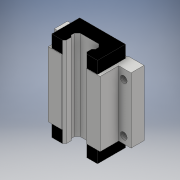
# Autodesk Inventor part: PATINS TRILHO LINEAR 15MM DFH-A_AL
Saved by Autodesk Inventor 2018 (Build 220112000, 112)
## iProperties
Created: 2018-09-22
Part Number: PATINS TRILHO LINEAR 15MM DFH-A_AL
Material: Genérico
Document SubType Name: Modeling
Designer: Usuario
Density: 1 g/cm^3
Appearance: Padrão
Author: Usuario
Autodesk Inventor part; units mm, degrees
ref_plane "YZ Plane" through (0, 0, 0) normal (1, 0, 0) x (0, 1, 0)
ref_plane "XZ Plane" through (0, 0, 0) normal (0, 1, 0) x (-1, 0, 0)
ref_plane "XY Plane" through (0, 0, 0) normal (0, 0, 1) x (1, 0, 0)
sketch "Esboço1" plane through (0, 0, 0) normal (0, 0, 1) x (1, 0, 0)
  line L0 (1.0341, 28.7122) -> (1.0341, -32.1101) construction
  line L1 (1.0341, 7.7011) -> (-4.7241, 7.7011)
  line L2 (-4.7241, 7.7011) -> (-6.4659, 5.9592)
  line L3 (-6.4659, 5.9592) -> (-6.4659, 3.9592)
  line L4 (-6.4659, 3.9592) -> (-5.2631, 2.7564)
  line L5 (-5.2631, 2.7564) -> (-5.2631, -0.2436)
  line L6 (-5.2631, -0.2436) -> (-6.4659, -1.4465)
  line L7 (-6.4659, -1.4465) -> (-6.4659, -1.6989)
  line L8 (-6.4659, -6.2989) -> (1.0341, -6.2989) construction
  line L9 (-22.4659, 9.7011) -> (-22.4659, 17.7011)
  line L10 (-17.9659, 24.9392) -> (-17.9659, -12.707) construction
  line L11 (-20.4659, 24.9392) -> (-20.4659, -12.707) construction
  line L12 (-15.4659, 24.9392) -> (-15.4659, -12.9196) construction
  line L13 (1.0341, 9.7011) -> (-29.6062, 9.7011) construction
  line L14 (-22.4659, 9.7011) -> (-14.8619, 9.7011)
  line L15 (-14.8619, 9.7011) -> (-14.8619, -1.6989)
  line L16 (1.0341, 16.4633) -> (-13.4863, 16.4633) construction
  line L17 (-13.4863, 16.4633) -> (-13.4863, -1.6989) construction
  arc A0 (-14.8619, -1.6989) -> (-22.4659, 9.7011) centre (-28.6186, -2.6389) ccw construction
  line L18 (-6.4659, -1.6989) -> (-6.4659, -6.2989) construction
  line L19 (-6.4659, -1.6989) -> (-14.8619, -1.6989)
  line L20 (-13.4863, 17.7011) -> (-12.9262, 17.1409)
  line L21 (-12.9262, 17.1409) -> (-5.8645, 17.1409)
  line L22 (-5.8645, 17.1409) -> (-5.3043, 17.7011)
  line L23 (-22.4659, 17.7011) -> (-13.4863, 17.7011)
  line L24 (-5.3043, 17.7011) -> (1.0341, 17.7011)
  line L25 (1.0341, 7.7011) -> (6.7923, 7.7011)
  line L26 (6.7923, 7.7011) -> (8.5341, 5.9592)
  line L27 (8.5341, 5.9592) -> (8.5341, 3.9592)
  line L28 (8.5341, 3.9592) -> (7.3313, 2.7564)
  line L29 (7.3313, 2.7564) -> (7.3313, -0.2436)
  line L30 (7.3313, -0.2436) -> (8.5341, -1.4465)
  line L31 (8.5341, -1.4465) -> (8.5341, -1.6989)
  line L32 (8.5341, -6.2989) -> (1.0341, -6.2989) construction
  line L33 (24.5341, 9.7011) -> (24.5341, 17.7011)
  line L34 (20.0341, 24.9392) -> (20.0341, -12.707) construction
  line L35 (22.5341, 24.9392) -> (22.5341, -12.707) construction
  line L36 (17.5341, 24.9392) -> (17.5341, -12.9196) construction
  line L37 (1.0341, 9.7011) -> (31.6744, 9.7011) construction
  line L38 (24.5341, 9.7011) -> (16.9301, 9.7011)
  line L39 (16.9301, 9.7011) -> (16.9301, -1.6989)
  line L40 (1.0341, 16.4633) -> (15.5546, 16.4633) construction
  line L41 (15.5546, 16.4633) -> (15.5546, -1.6989) construction
  arc A1 (24.5341, 9.7011) -> (16.9301, -1.6989) centre (30.6868, -2.6389) ccw construction
  line L42 (8.5341, -1.6989) -> (8.5341, -6.2989) construction
  line L43 (8.5341, -1.6989) -> (16.9301, -1.6989)
  line L44 (15.5546, 17.7011) -> (14.9944, 17.1409)
  line L45 (14.9944, 17.1409) -> (7.9327, 17.1409)
  line L46 (7.9327, 17.1409) -> (7.3725, 17.7011)
  line L47 (24.5341, 17.7011) -> (15.5546, 17.7011)
  line L48 (7.3725, 17.7011) -> (1.0341, 17.7011)
  dimension "d11" = 45
  dimension "d12" = 3
  dimension "d13" = 14
  dimension "d14" = 2
  dimension "d15" = 7.5
  dimension "d19" = 23.5
  dimension "d21" = 2.5
  dimension "d22" = 2.5
  dimension "d23" = 19
  constraints: 98 end point, 26 symmetric about line, 15 point on line, 9 perpendicular, 5 horizontal, 5 vertical, 4 point on circle, 2 centre point, 2 parallel, 1 other
  measures "d11" angle of L2 L1
  measures "d12" distance of L4.end L5.end
  measures "d13" distance between parallel lines of L8 L1
  measures "d14" distance of L2.end L3.end
  measures "d15" distance of L8.start L8.end
  measures "d19" distance of L9.end L24.end
  measures "d21" distance between parallel lines of L12 L10
  measures "d22" distance between parallel lines of L10 L11
  measures "d23" distance between parallel lines of L10 L0
extrude "Extrusão2" add sketch "Esboço1" along normal blind 40
sketch "Esboço2" plane through (0, 0, 40) normal (0, 0, 1) x (1, 0, 0)
  line L0 (-13.0314, -1.4465) -> (-13.0314, 15.7348)
  line L1 (-13.0314, 15.7348) -> (15.0996, 15.7348)
  line L2 (15.0996, 15.7348) -> (15.0996, -1.4465)
  line L3 (-6.4659, -1.4465) -> (-5.2631, -0.2436) projected
  line L4 (-6.4659, -1.4465) -> (-5.2631, -0.2436)
  line L5 (-5.2631, 2.7564) -> (-6.4659, 3.9592) projected
  line L6 (-5.2631, -0.2436) -> (-5.2631, 2.7564)
  line L7 (-5.2631, 2.7564) -> (-6.4659, 3.9592)
  line L8 (-6.4659, 3.9592) -> (-6.4659, 5.9592) projected
  line L9 (-6.4659, 3.9592) -> (-6.4659, 5.9592)
  line L10 (-6.4659, 5.9592) -> (-4.7241, 7.7011) projected
  line L11 (-6.4659, 5.9592) -> (-4.7241, 7.7011)
  line L12 (-4.7241, 7.7011) -> (6.7923, 7.7011) projected
  line L13 (-4.7241, 7.7011) -> (6.7923, 7.7011)
  line L14 (6.7923, 7.7011) -> (8.5341, 5.9592) projected
  line L15 (6.7923, 7.7011) -> (8.5341, 5.9592)
  line L16 (8.5341, 3.9592) -> (8.5341, 5.9592) projected
  line L17 (8.5341, 5.9592) -> (8.5341, 3.9592)
  line L18 (7.3313, -0.2436) -> (7.3313, 2.7564) projected
  line L19 (8.5341, 3.9592) -> (7.3313, 2.7564)
  line L20 (7.3313, 2.7564) -> (7.3313, -0.2436)
  line L21 (8.5341, -1.4465) -> (7.3313, -0.2436) projected
  line L22 (7.3313, -0.2436) -> (8.5341, -1.4465)
  line L23 (15.0996, -1.4465) -> (8.5341, -1.4465)
  line L24 (-6.4659, -1.4465) -> (-13.0314, -1.4465)
  constraints: 32 end point, 7 collinear, 4 parallel, 2 horizontal, 2 perpendicular, 1 vertical
extrude "Extrusão3" add sketch "Esboço2" along normal blind 7.5
sketch "Esboço3" plane through (0, 0, 0) normal (0, 0, -1) x (-1, 0, 0)
  line L0 (-15.0996, -1.4465) -> (-15.0996, 15.7348)
  line L1 (-15.0996, 15.7348) -> (13.0314, 15.7348)
  line L2 (13.0314, 15.7348) -> (13.0314, -1.4465)
  line L3 (-8.5341, -1.4465) -> (-7.3313, -0.2436)
  line L4 (-8.5341, -1.4465) -> (-7.3313, -0.2436)
  line L5 (-7.3313, 2.7564) -> (-8.5341, 3.9592)
  line L6 (-7.3313, -0.2436) -> (-7.3313, 2.7564)
  line L7 (-7.3313, 2.7564) -> (-8.5341, 3.9592)
  line L8 (-8.5341, 3.9592) -> (-8.5341, 5.9592)
  line L9 (-8.5341, 3.9592) -> (-8.5341, 5.9592)
  line L10 (-8.5341, 5.9592) -> (-6.7923, 7.7011)
  line L11 (-8.5341, 5.9592) -> (-6.7923, 7.7011)
  line L12 (-6.7923, 7.7011) -> (4.7241, 7.7011)
  line L13 (-6.7923, 7.7011) -> (4.7241, 7.7011)
  line L14 (4.7241, 7.7011) -> (6.4659, 5.9592)
  line L15 (4.7241, 7.7011) -> (6.4659, 5.9592)
  line L16 (6.4659, 3.9592) -> (6.4659, 5.9592)
  line L17 (6.4659, 5.9592) -> (6.4659, 3.9592)
  line L18 (5.2631, -0.2436) -> (5.2631, 2.7564)
  line L19 (6.4659, 3.9592) -> (5.2631, 2.7564)
  line L20 (5.2631, 2.7564) -> (5.2631, -0.2436)
  line L21 (6.4659, -1.4465) -> (5.2631, -0.2436)
  line L22 (5.2631, -0.2436) -> (6.4659, -1.4465)
  line L23 (13.0314, -1.4465) -> (6.4659, -1.4465)
  line L24 (-8.5341, -1.4465) -> (-15.0996, -1.4465)
  point P0 (0, 0)
  point P1 (-1.0341, 15.7348)
  constraints: 50 end point, 7 collinear, 4 parallel, 2 horizontal, 2 perpendicular, 1 midpoint, 1 vertical
extrude "Extrusão4" add sketch "Esboço3" along normal blind 7.5
sketch "Esboço4" plane through (-5.3043, 17.7011, 0) normal (0, 1, 0) x (1, 0, 0)
  line L0 (6.3384, -52.3357) -> (6.3384, 13.624) construction
  line L1 (-22.2826, -19.2901) -> (34.758, -19.2901) construction
  circle A0 centre (-12.6616, -34.2901) radius 1 construction
  circle A1 centre (-12.6616, -4.2901) radius 1 construction
  circle A2 centre (25.3384, -34.2901) radius 1 construction
  circle A3 centre (25.3384, -4.2901) radius 1 construction
  dimension "d31" = 2
  dimension "d32" = 2
  dimension "d33" = 2
  dimension "d34" = 2
  dimension "d35" = 19
  dimension "d36" = 19
  dimension "d37" = 19
  dimension "d38" = 19
  dimension "d39" = 15
  dimension "d40" = 15
  dimension "d41" = 15
  dimension "d42" = 15
  constraints: 4 centre point, 4 end point, 1 horizontal, 1 vertical
  measures "d31" diameter of A0
  measures "d32" diameter of A1
  measures "d33" diameter of A2
  measures "d34" diameter of A3
  measures "d35" distance from line of L0 A0.centre
  measures "d36" distance from line of L0 A2.centre
  measures "d37" distance from line of L0 A1.centre
  measures "d38" distance from line of L0 A3.centre
  measures "d39" distance from line of A1.centre L1
  measures "d40" distance from line of A0.centre L1
  measures "d41" distance from line of L1 A3.centre
  measures "d42" distance from line of A2.centre L1
hole "Furo1" at (-17.9659, 17.7011, 4.2901) at (-17.9659, 17.7011, 34.2901) at (20.0341, 17.7011, 34.2901) at (20.0341, 17.7011, 4.2901) direction (0, -1, 0) diameter 4.134 end through all thread size "M5x0.8" class "6H" standard "ANSI Metric M Profile"
equation "\"d22\" = d21"
equation "\"d36\" = d35"
equation "\"d37\" = d35"
equation "\"d38\" = d35"
equation "\"d40\" = d39"
equation "\"d41\" = d39"
equation "\"d42\" = d39"
